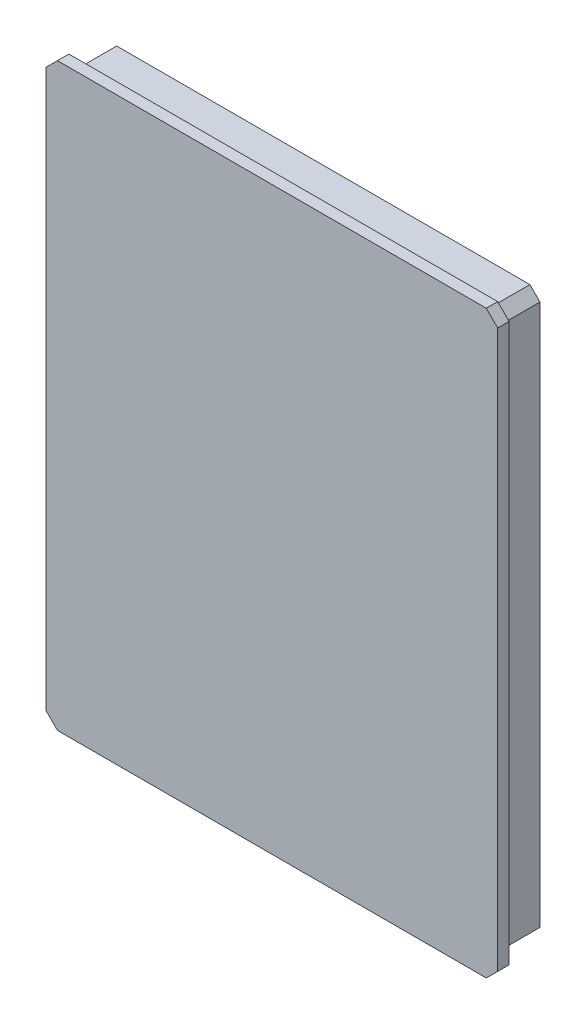
# Autodesk Inventor part: CaseButtom
Saved by Autodesk Inventor 2025.2 (Build 292293000, 293)
## iProperties
Created: 2026-02-20
Part Number: CaseButtom
Material: 一般
Document SubType Name: Modeling
Designer: naka6
Density: 1 g/cm^3
Appearance: 既定
Author: naka6
Autodesk Inventor part; units mm, degrees
ref_plane "YZ Plane" through (0, 0, 0) normal (1, 0, 0) x (0, 1, 0)
ref_plane "XZ Plane" through (0, 0, 0) normal (0, 1, 0) x (-1, 0, 0)
ref_plane "XY Plane" through (0, 0, 0) normal (0, 0, 1) x (1, 0, 0)
sketch "スケッチ2" plane through (0, 0, 0) normal (0, 0, 1) x (1, 0, 0)
  line L0 (-18.1069, 29.75) -> (19.4146, 29.75) projected
  line L1 (-19.1069, 28.75) -> (-18.1069, 29.75) projected
  line L2 (-19.1069, -20) -> (-19.1069, 28.75) projected
  line L3 (-17.5069, 29.15) -> (18.8146, 29.15) projected
  line L4 (19.8146, 28.15) -> (18.8146, 29.15) projected
  line L5 (19.8146, 28.15) -> (19.8146, -19.4) projected
  line L6 (18.8146, -20.4) -> (19.8146, -19.4) projected
  line L7 (18.8146, -20.4) -> (-17.5069, -20.4) projected
  line L8 (-18.5069, -19.4) -> (-17.5069, -20.4) projected
  line L9 (-18.5069, -19.4) -> (-18.5069, 28.15) projected
  line L10 (-17.5069, 29.15) -> (-18.5069, 28.15) projected
  line L11 (-19.1069, 28.75) -> (-18.1069, 29.75) projected
  line L12 (-19.1069, -20) -> (-19.1069, 28.75) projected
  line L13 (-18.1069, -21) -> (-19.1069, -20) projected
  line L14 (19.4146, -21) -> (-18.1069, -21) projected
  line L15 (20.4146, -20) -> (19.4146, -21) projected
  line L16 (20.4146, 28.75) -> (20.4146, -20) projected
  line L17 (19.4146, 29.75) -> (20.4146, 28.75) projected
  line L18 (-18.1069, 29.75) -> (19.4146, 29.75) projected
  line L19 (18.7318, 28.95) -> (-17.424, 28.95)
  line L20 (-17.424, 28.95) -> (-18.3069, 28.0672)
  line L21 (-18.3069, 28.0672) -> (-18.3069, -19.3172)
  line L22 (-18.3069, -19.3172) -> (-17.424, -20.2)
  line L23 (-17.424, -20.2) -> (18.7318, -20.2)
  line L24 (18.7318, -20.2) -> (19.6146, -19.3172)
  line L25 (19.6146, -19.3172) -> (19.6146, 28.0672)
  line L26 (19.6146, 28.0672) -> (18.7318, 28.95)
  line L27 (-17.1341, 28.25) -> (18.4418, 28.25)
  line L28 (18.4418, 28.25) -> (18.9146, 27.7772)
  line L29 (18.9146, 27.7772) -> (18.9146, -19.0272)
  line L30 (18.9146, -19.0272) -> (18.4418, -19.5)
  line L31 (18.4418, -19.5) -> (-17.1341, -19.5)
  line L32 (-17.1341, -19.5) -> (-17.6069, -19.0272)
  line L33 (-17.6069, -19.0272) -> (-17.6069, 27.7772)
  line L34 (-17.6069, 27.7772) -> (-17.1341, 28.25)
  point P0 (0, 0)
  dimension "d0" = 0.2
  dimension "d1" = 0.7
  constraints: 32 end point, 15 other
  measures "d0" distance between parallel lines of L3 L19
  measures "d1" distance between parallel lines of L19 L27
extrude "押し出し1" add sketch "スケッチ2" against normal blind 3.5 contours L26 L25 L24 L23 L22 L21 L20 L19
sketch "スケッチ3" plane through (0, 0, 0) normal (0, 0, 1) x (1, 0, 0)
  line L0 (-17.5069, 29.15) -> (18.8146, 29.15) projected
  line L1 (19.8146, 28.15) -> (18.8146, 29.15) projected
  line L2 (19.8146, 28.15) -> (19.8146, -19.4) projected
  line L3 (18.8146, -20.4) -> (19.8146, -19.4) projected
  line L4 (18.8146, -20.4) -> (-17.5069, -20.4) projected
  line L5 (-18.5069, -19.4) -> (-17.5069, -20.4) projected
  line L6 (-18.5069, -19.4) -> (-18.5069, 28.15) projected
  line L7 (-17.5069, 29.15) -> (-18.5069, 28.15) projected
  line L8 (-19.1069, 28.75) -> (-18.1069, 29.75) projected
  line L9 (-19.1069, -20) -> (-19.1069, 28.75) projected
  line L10 (-18.1069, -21) -> (-19.1069, -20) projected
  line L11 (19.4146, -21) -> (-18.1069, -21) projected
  line L12 (20.4146, -20) -> (19.4146, -21) projected
  line L13 (20.4146, 28.75) -> (20.4146, -20) projected
  line L14 (19.4146, 29.75) -> (20.4146, 28.75) projected
  line L15 (-18.1069, 29.75) -> (19.4146, 29.75) projected
  point P0 (0, 0)
extrude "押し出し2" add sketch "スケッチ3" along normal blind 1 contours L0 L1 L2 L3 L4 L5 L6 L7 | L8 L15 L14 L13 L12 L11 L10 L9
